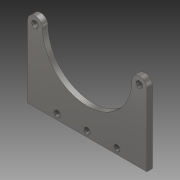
# Autodesk Inventor part: motor_end_plate
Saved by Autodesk Inventor 2019 (Build 230136000, 136)
## iProperties
Created: 2018-09-24
Part Number: motor_end_plate
Material: Steel, Mild
Document SubType Name: Modeling
Designer: Callum Snowden
Mass: 175.009 g
Surface Area: 114.035 cm^2
Volume: 22.2941 cm^3
Density: 7.85 g/cm^3
Appearance: Semi-Polished
Author: Callum Snowden
Autodesk Inventor part; units mm, degrees
ref_plane "YZ Plane" through (0, 0, 0) normal (1, 0, 0) x (0, 1, 0)
ref_plane "XZ Plane" through (0, 0, 0) normal (0, 1, 0) x (-1, 0, 0)
ref_plane "XY Plane" through (0, 0, 0) normal (0, 0, 1) x (1, 0, 0)
sketch "Sketch1" plane through (0, 0, 0) normal (0, 0, 1) x (1, 0, 0)
  line L0 (-75.6, 0) -> (75.6, 0) construction
  line L1 (0, 21.1) -> (0, -79.35) construction
  line L2 (54, 0) -> (54, -65)
  line L3 (54, -65) -> (-54, -65)
  line L4 (-54, -65) -> (-54, 0)
  circle A0 centre (47.25, 0) radius 3
  circle A1 centre (-47.25, 0) radius 3
  arc A2 (-40.5, 0) -> (-54, 0) centre (-47.25, 0) ccw
  arc A3 (54, 0) -> (40.5, 0) centre (47.25, 0) ccw
  arc A4 (-40.5, 0) -> (40.5, 0) centre (0, 0) ccw
  dimension "d0" = 108
  dimension "d2" = 6
  dimension "d3" = 6
  dimension "d6" = 94.5
  dimension "d9" = 65
  constraints: 6 end point, 6 point on circle, 5 centre point, 4 tangent, 2 coincident, 2 parallel, 2 point on line, 1 line through centre, 1 symmetric about line, 1 other
  measures "d0" distance of L2.end L3.end
  measures "d2" diameter of A0
  measures "d3" diameter of A1
  measures "d6" distance of A1.centre A0.centre
  measures "d9" distance of L3.end L4.end
extrude "Extrusion1" add sketch "Sketch1" along normal blind 5
sketch "Sketch2" plane through (0, 0, 5) normal (0, 0, 1) x (1, 0, 0)
  circle A0 centre (-47.25, 0) radius 3 construction
  circle A1 centre (47.25, 0) radius 3 construction
  line L0 (54, -65) -> (54, 0) construction
  arc A2 (54, 0) -> (40.5, 0) centre (47.25, 0) ccw construction
  arc A3 (-40.5, 0) -> (40.5, 0) centre (0, 0) ccw construction
  arc A4 (-40.5, 0) -> (-54, 0) centre (-47.25, 0) ccw construction
  line L1 (-54, 0) -> (-54, -65) construction
  line L2 (-54, -65) -> (54, -65) construction
  line L3 (-54, -60) -> (54, -60) construction
  line L4 (54, -65) -> (54, 0) construction
  line L5 (0, 21.1) -> (0, -79.35) construction
  point P0 (27, -60)
  point P1 (-27, -60)
  point P2 (0, -60)
  dimension "d12" = 5
  dimension "d13" = 54
  constraints: 5 point on line, 2 end point, 1 midpoint, 1 perpendicular, 1 symmetric about line
  measures "d12" distance between parallel lines of L2 L3
  measures "d13" distance of point (27, -60) point (-27, -60)
hole "Hole1" at (27, -60, 5) at (-27, -60, 5) at (0, -60, 5) direction (0, 0, -1) diameter 5.5 end through all
body "Solid1"
